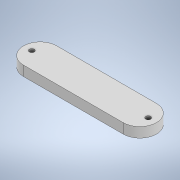
# Autodesk Inventor part: fuselagewingconnection
Saved by Autodesk Inventor 2022 (Build 260153000, 153)
## iProperties
Created: 2021-08-25
Part Number: fuselagewingconnection
Material: Generic
Document SubType Name: Modeling
Designer: Ferdinand Hubbard
Density: 1 g/cm^3
Appearance: Default
Author: Ferdinand Hubbard
Autodesk Inventor part; units mm, degrees
ref_plane "YZ Plane" through (0, 0, 0) normal (1, 0, 0) x (0, 1, 0)
ref_plane "XZ Plane" through (0, 0, 0) normal (0, 1, 0) x (-1, 0, 0)
ref_plane "XY Plane" through (0, 0, 0) normal (0, 0, 1) x (1, 0, 0)
sketch "Sketch1" plane through (0, 0, 0) normal (0, 1, 0) x (-1, 0, 0)
  line L0 (30, -10) -> (-30, -10)
  line L1 (-40, 0) -> (-40, 0)
  line L2 (-30, 10) -> (30, 10)
  line L3 (40, 0) -> (40, 0)
  line L4 (40, -10) -> (-40, 10) construction
  line L5 (-40, -10) -> (40, 10) construction
  line L6 (0, 0) -> (35, 0)
  line L7 (0, 0) -> (35, 0) construction
  line L8 (0, 0) -> (-35, 0) construction
  line L9 (0, 0) -> (35, 0) construction
  circle A0 centre (35, 0) radius 1.5
  circle A1 centre (-35, 0) radius 1.5
  arc A2 (-30, 10) -> (-40, 0) centre (-30, 0) ccw
  arc A3 (-40, 0) -> (-30, -10) centre (-30, 0) ccw
  arc A4 (30, -10) -> (40, 0) centre (30, 0) ccw
  arc A5 (40, 0) -> (30, 10) centre (30, 0) ccw
  point P0 (40, 0)
  point P1 (-40, 0)
  dimension "d0" = 80
  dimension "d1" = 20
  dimension "d3" = 35
  dimension "d4" = 0
  dimension "d5" = 35
  dimension "d6" = 180
  dimension "d7" = 3
  dimension "d8" = 3
  dimension "d11" = 10
  constraints: 20 end point, 8 point on circle, 8 point on line, 8 tangent, 6 centre point, 4 horizontal, 3 equal length, 3 equal radius, 2 coincident, 2 collinear, 2 midpoint, 1 perpendicular
  measures "d0" distance of L4.end L5.end
  measures "d1" distance of L5.start L4.end
  measures "d3" distance of L6.start L6.end
  measures "d4" distance between parallel lines of L6 L7
  measures "d5" distance of L6.start L8.end
  measures "d6" angle of L8 L9
  measures "d7" diameter of A0
  measures "d8" diameter of A1
  measures "d11" radius of A2
extrude "Extrusion1" add sketch "Sketch1" along normal blind 6
body "Solid1"
